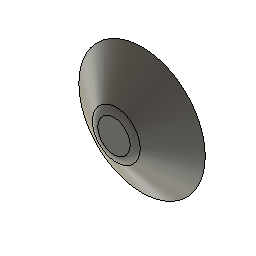
_Bolt Ramp Cover.b14d74ff-13b3-4bcc-bf03-41ef3c5aef0e (Autodesk Fusion 360 design; units mm, degrees)
Autodesk Fusion 360 part; units mm, degrees
sketch "Sketch1" plane through (0, 0, 0) normal (0, 1, 0) x (1, 0, 0)
  circle A0 centre (0, 0) radius 5.25
  circle A1 centre (0, 0) radius 7.25
  dimension "d1" = 10.5
  dimension "d2" = 2
  constraint coincident A0.centre A1.centre
  measures "d1" diameter of A0
extrude "Extrude1" add sketch "Sketch1" along normal blind 6
sketch "Sketch2" plane through (0, 0, 0) normal (0, -1, 0) x (1, 0, 0)
  circle A0 centre (0, 0) radius 5.25
  circle A1 centre (0, 0) radius 7.25
  circle A2 centre (0, 0) radius 7.25
extrude "Extrude2" add sketch "Sketch2" along normal blind 4 contours A0 | A1 A2
sketch "Sketch3" plane through (0, 6, 0) normal (0, 1, 0) x (-1, 0, 0)
  circle A0 centre (0, 0) radius 5.25
  circle A1 centre (0, 0) radius 7.25
  circle A2 centre (0, 0) radius 7.25
  circle A3 centre (0, 0) radius 22.5
  dimension "d7" = 45
  constraint concentric A2 A3
  measures "d7" diameter of A3
loft "Loft1" add profiles "Sketch3" section 1 contours A3 section 2 face at (1.965, -4, -0.3602)
sketch "Sketch4" plane through (0, 6, 0) normal (0, 1, 0) x (-1, 0, 0)
  circle A0 centre (0, 0) radius 22.5
  circle A1 centre (0, 0) radius 4.875 construction
  circle A2 centre (0, 0) radius 6
  line L0 (0, 0) -> (0, -6) construction
  line L1 (-0.75, -6) -> (0.75, -6)
  line L2 (0.75, -6) -> (0.75, -4.875)
  line L3 (0.75, -4.875) -> (-0.75, -4.875)
  line L4 (-0.75, -4.875) -> (-0.75, -6)
  line L5 (-0.75, -6) -> (0.75, -4.875) construction
  line L6 (0.75, -6) -> (-0.75, -4.875) construction
  line L7 (5.5712, -2.3505) -> (4.5969, -1.788)
  line L8 (4.5969, -1.788) -> (3.8469, -3.087)
  line L9 (3.8469, -3.087) -> (4.8212, -3.6495)
  line L10 (4.8212, -3.6495) -> (5.5712, -2.3505)
  line L11 (4.8212, 3.6495) -> (3.8469, 3.087)
  line L12 (3.8469, 3.087) -> (4.5969, 1.788)
  line L13 (4.5969, 1.788) -> (5.5712, 2.3505)
  line L14 (5.5712, 2.3505) -> (4.8212, 3.6495)
  line L15 (-0.75, 6) -> (-0.75, 4.875)
  line L16 (-0.75, 4.875) -> (0.75, 4.875)
  line L17 (0.75, 4.875) -> (0.75, 6)
  line L18 (0.75, 6) -> (-0.75, 6)
  line L19 (-5.5712, 2.3505) -> (-4.5969, 1.788)
  line L20 (-4.5969, 1.788) -> (-3.8469, 3.087)
  line L21 (-3.8469, 3.087) -> (-4.8212, 3.6495)
  line L22 (-4.8212, 3.6495) -> (-5.5712, 2.3505)
  line L23 (-4.8212, -3.6495) -> (-3.8469, -3.087)
  line L24 (-3.8469, -3.087) -> (-4.5969, -1.788)
  line L25 (-4.5969, -1.788) -> (-5.5712, -2.3505)
  line L26 (-5.5712, -2.3505) -> (-4.8212, -3.6495)
  point P0 (0, -5.4375)
  dimension "d8" = 9.75
  dimension "d9" = 12
  dimension "d10" = 1.5
  dimension "d12" = 360
  constraint coincident A0.centre A1.centre
  constraint coincident A2 L0.end
  constraint vertical L0
  constraint horizontal L1
  constraint perpendicular L1 L2
  constraint parallel L1 L3
  constraint parallel L2 L4
  constraint coincident L5 P0
  constraint coincident L6 P0
  constraint coincident L0 P0
  constraint tangent A1 L3
  constraint coincident L0.end L1
  measures "d8" diameter of A1
  measures "d9" diameter of A2
  measures "d10" distance of L2.end L3.end
extrude "Extrude3" cut sketch "Sketch4" against normal blind 8 contours A2 L2 L3 L4 L7 L8 L9 L11 L12 L13 L15 L16 L17 L19 L20 L21 L23 L24 L25
fillet "Fillet1" radius 5 1 edges at (-6.7594, -4, -2.6217)
